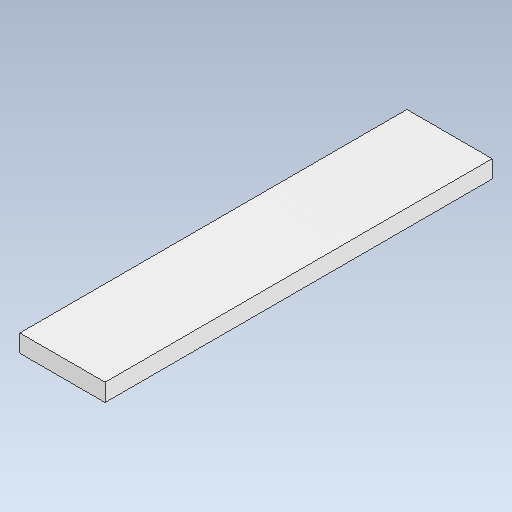
# Autodesk Inventor part: Part8
Saved by Autodesk Inventor 2021 (Build 250183000, 183)
## iProperties
Created: 2021-07-03
Part Number: Part8
Material: LCP Plastic
Document SubType Name: Modeling
Designer: VK
Density: 1.626 g/cm^3
Appearance: Smooth - White
Author: VK
Autodesk Inventor part; units mm, degrees
ref_plane "YZ Plane" through (0, 0, 0) normal (1, 0, 0) x (0, 1, 0)
ref_plane "XZ Plane" through (0, 0, 0) normal (0, 1, 0) x (-1, 0, 0)
ref_plane "XY Plane" through (0, 0, 0) normal (0, 0, 1) x (1, 0, 0)
sketch "Sketch1" plane through (0, 0, 0) normal (0, 1, 0) x (-1, 0, 0)
  line L0 (0, 0) -> (24.226, 0)
  line L1 (24.226, 0) -> (24.226, -110)
  line L2 (24.226, -110) -> (0, -110)
  line L3 (0, -110) -> (0, 0)
  dimension "d0" = 24.226
  dimension "d1" = 110
  constraints: 8 end point, 2 parallel, 1 horizontal, 1 perpendicular
  measures "d0" distance of L1.end L2.end
  measures "d1" distance of L0.end L1.end
extrude "Extrusion1" add sketch "Sketch1" along normal blind 5
body "Solid1"
